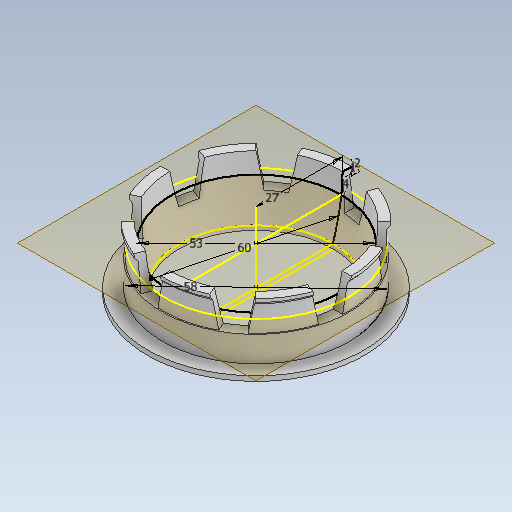
# Autodesk Inventor part: motor_frontalholder
Saved by Autodesk Inventor 2020 (Build 240168000, 168)
## iProperties
Created: 2019-08-02
Part Number: motor_frontalholder
Material: Generic
Document SubType Name: Modeling
Designer: erwin
Density: 1 g/cm^3
Appearance: Default
Mass: 11.323 g
Surface Area: 92.4119 cm^2
Volume: 11.323 cm^3
Author: erwin
Autodesk Inventor part; units mm, degrees
ref_plane "YZ Plane" through (0, 0, 0) normal (1, 0, 0) x (0, 1, 0)
ref_plane "XZ Plane" through (0, 0, 0) normal (0, 1, 0) x (-1, 0, 0)
ref_plane "XY Plane" through (0, 0, 0) normal (0, 0, 1) x (1, 0, 0)
sketch "Sketch1" plane through (0, 0, 0) normal (0, 1, 0) x (-1, 0, 0)
  circle A0 centre (0, 0) radius 34
  circle A1 centre (0, 0) radius 24
  dimension "d1" = 68
  dimension "d2" = 48
  constraints: 2 centre point, 1 coincident
  measures "d1" diameter of A0
  measures "d2" diameter of A1
sketch "Sketch1 outline for Extrusion1" plane through (0, 0, 0) normal (0, 1, 0) x (-1, 0, 0)
  circle A0 centre (0, 0) radius 34
  circle A1 centre (0, 0) radius 24
extrude "Extrusion1" add sketch "Sketch1 outline for Extrusion1" along normal blind 1.5
sketch "Sketch2" plane through (0, 1.5, 0) normal (0, 1, 0) x (1, 0, 0)
  circle A0 centre (0, 0) radius 24 projected
  circle A1 centre (0, 0) radius 29
  dimension "d5" = 58
  constraints: 1 centre point, 1 coincident
  measures "d5" diameter of A1
ref_plane "Work Plane1" through (0, 13.5, 0) normal (0, 1, 0) x (1, 0, 0)
sketch "Sketch3" plane through (0, 13.5, 0) normal (0, 1, 0) x (1, 0, 0)
  circle A0 centre (0, 0) radius 29 projected
  circle A1 centre (0, 0) radius 26.5
  dimension "d7" = 53
  constraints: 1 centre point, 1 coincident
  measures "d7" diameter of A1
sketch "Sketch4" plane through (0, 0, 0) normal (1, 0, 0) x (0, 1, 0)
  line L0 (13.5, -26.5) -> (13.5, 26.5)
  line L1 (1.5, 24) -> (1.5, -24)
  line L2 (0, 24) -> (0, -24)
  line L3 (1.5, 24) -> (1.5, -24)
  arc A0 (1.5, -24) -> (19.5, -27) centre (20.24922, 32.995322) ccw
  line L4 (1.5, -29) -> (1.5, 29)
  line L5 (13.5, -29) -> (13.5, 29)
  line L6 (13.5, -29) -> (1.5, -29)
  line L7 (-3.934649, 0) -> (23.607895, 0)
  line L8 (13.5, -29) -> (17.5, -29)
  line L9 (17.5, -29) -> (18.5, -29.874686)
  line L10 (19.5, -29.874686) -> (19.5, -27)
  line L11 (19.5, -29.874686) -> (18.5, -29.874686)
  point P0 (0, 0)
  point P1 (13.5, -26.62387)
  dimension "d8" = 60
  dimension "d12" = 4
  dimension "d13" = 2
  dimension "d14" = 1
  dimension "d20" = 27
  constraints: 10 end point, 3 horizontal, 2 point on circle, 1 centre point, 1 perpendicular
  measures "d8" radius of A0
  measures "d12" distance of L5.start L8.end
  measures "d13" distance from line of L10 L8.end
  measures "d14" distance of L10.start L9.end
  measures "d20" distance from line of L7 L10.end
sketch "Sketch4 outline for Revolution1" plane through (0, 0, 0) normal (1, 0, 0) x (0, 1, 0)
  line L0 (1.5, -24) -> (1.5, -29)
  arc A0 (19.5, -27) -> (1.5, -24) centre (20.24922, 32.995322) cw
  line L1 (19.5, -29.874686) -> (19.5, -27)
  line L2 (18.5, -29.874686) -> (19.5, -29.874686)
  line L3 (17.5, -29) -> (18.5, -29.874686)
  line L4 (13.5, -29) -> (17.5, -29)
  line L5 (1.5, -29) -> (13.5, -29)
revolve "Revolution1" add sketch "Sketch4 outline for Revolution1" angle 360 about axis through (0, -10, 0) along (0, 1, 0)
sketch "Sketch5" plane through (0, 0, 0) normal (1, 0, 0) x (0, 1, 0)
  line L0 (0, 34) -> (1.5, 34)
  line L1 (1.5, 34) -> (1.5, 29)
  line L2 (1.5, 29) -> (17.5, 29)
  line L3 (17.5, 29) -> (18.5, 29.874686)
  line L4 (18.5, 29.874686) -> (19.5, 29.874686)
  line L5 (19.5, 29.874686) -> (19.5, 27)
  arc A0 (19.5, 27) -> (1.5, 24) centre (20.24922, -32.995322) ccw
  line L6 (1.5, 24) -> (0, 24)
  line L7 (0, 24) -> (0, 34)
  line L8 (1.5, -34) -> (0, -34)
  line L9 (0, -34) -> (0, -24)
  line L10 (0, -24) -> (1.5, -24)
  arc A1 (1.5, -24) -> (19.5, -27) centre (20.24922, 32.995322) ccw
  line L11 (19.5, -27) -> (19.5, -29.874686)
  line L12 (19.5, -29.874686) -> (18.5, -29.874686)
  line L13 (18.5, -29.874686) -> (17.5, -29)
  line L14 (17.5, -29) -> (1.5, -29)
  line L15 (1.5, -29) -> (1.5, -34)
  line L16 (17.5, 29) -> (1.5, 29)
  line L17 (9.5, 29) -> (9.5, 26.033944)
  point P0 (0, 0)
  constraints: 2 end point, 1 midpoint, 1 perpendicular, 1 point on circle
sketch "Sketch5 outline for Revolution2" plane through (0, 0, 0) normal (1, 0, 0) x (0, 1, 0)
  line L0 (19.5, 27) -> (19.5, 29.874686)
  arc A0 (9.5, 26.033944) -> (19.5, 27) centre (20.24922, -32.995322) cw
  line L1 (9.5, 29) -> (9.5, 26.033944)
  line L2 (17.5, 29) -> (9.5, 29)
  line L3 (18.5, 29.874686) -> (17.5, 29)
  line L4 (19.5, 29.874686) -> (18.5, 29.874686)
revolve "Revolution2" cut sketch "Sketch5 outline for Revolution2" angle 20 about axis through (0, -10, 0) along (0, -1, 0)
draft "FaceDraft1" angle 10 pull direction (0, 1, 0) faces at (-9.638374, 13.271198, 26.481214) (0, 13.271198, 28.180719) fixed edges at (-9.726144, 19.5, 26.722361) (0, 19.5, 28.437343)
pattern_circular "Circular Pattern1" count 8 over 360 about axis through (0, -10, 0) along (0, 1, 0) of "Revolution2", "FaceDraft1"
sketch "Sketch6" plane through (0, 1.5, 0) normal (0, 1, 0) x (1, 0, 0)
  circle A0 centre (0, 0) radius 29.375
  circle A1 centre (0, 0) radius 29 projected
  dimension "d21" = 58.75
  constraints: 1 centre point, 1 coincident
  measures "d21" diameter of A0
sketch "Sketch6 outline for Extrusion2" plane through (0, 1.5, 0) normal (0, 1, 0) x (1, 0, 0)
  circle A0 centre (0, 0) radius 29.375
  circle A1 centre (0, 0) radius 29
extrude "Extrusion2" add sketch "Sketch6 outline for Extrusion2" along normal up to surface (8 mm away)
body "Solid1"
